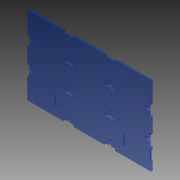
# Autodesk Inventor part: tableTop
Saved by Autodesk Inventor 2015 SP1 (Build 190203100, 203)
## iProperties
Created: 2015-04-09
Part Number: tableTop
Material: Generic
Document SubType Name: Modeling
Designer: Iain
Density: 1 g/cm^3
Appearance: Clear - Blue
Author: Iain
Autodesk Inventor part; units mm, degrees
(part 1 of 2)
sketch "Sketch1" plane through (0, 0, 0) normal (0, 1, 0) x (-1, 0, 0)
  line L0 (590, -375) -> (-590, -375)
  line L1 (-590, -375) -> (-590, 375)
  line L2 (-590, 375) -> (590, 375)
  line L3 (590, 375) -> (590, -375)
  point P0 (0, 0)
  point P1 (590, 0)
  point P2 (0, -375)
  dimension "d0" = 1180
  dimension "d1" = 750
  constraints: 8 end point, 2 midpoint, 2 parallel, 1 horizontal, 1 horizontal alignment, 1 perpendicular, 1 vertical alignment
  measures "d0" distance of L0.start L0.end
  measures "d1" distance of L2.end L0.start
extrude "Extrusion1" add sketch "Sketch1" along normal blind 18
sketch "Sketch2" plane through (0, 18, 0) normal (0, 1, 0) x (1, 0, 0)
  line L0 (590, 375) -> (-590, 375) projected
  line L1 (-590, 375) -> (-590, -375) projected
  line L2 (-590, -375) -> (590, -375) projected
  line L3 (590, -375) -> (590, 375) projected
  line L4 (-590, 175) -> (-572, 175)
  line L5 (-572, 175) -> (-572, 75)
  line L6 (-572, 75) -> (-590, 75)
  line L7 (-590, 75) -> (-590, 175)
  point P0 (0, 0)
  point P1 (-590, 125)
  point P2 (-590, 0)
  dimension "d4" = 18
  dimension "d5" = 100
  dimension "d6" = 250
  constraints: 8 end point, 2 midpoint, 2 parallel, 1 horizontal, 1 perpendicular, 1 vertical alignment
  measures "d4" distance of L4.start L4.end
  measures "d5" distance of L4.end L5.end
  measures "d6" distance of point (-590, 125) L0.end
extrude "Extrusion2" cut sketch "Sketch2" against normal blind 18 contours L4 L5 L6 L1
sketch "Sketch7" plane through (0, 18, 0) normal (0, 1, 0) x (1, 0, 0)
  line L0 (-590, 175) -> (-572, 175) projected
  line L1 (-572, 175) -> (-572, 75) projected
  line L2 (-572, 75) -> (-590, 75) projected
  line L3 (-590, 75) -> (-590, -375) projected
  line L4 (-590, -375) -> (590, -375) projected
  line L5 (590, -375) -> (590, 375) projected
  line L6 (590, 375) -> (-590, 375) projected
  line L7 (-590, 375) -> (-590, 175) projected
  line L8 (-590, 134) -> (-531, 134)
  line L9 (-531, 134) -> (-531, 116)
  line L10 (-531, 116) -> (-590, 116)
  line L11 (-590, 116) -> (-590, 134)
  point P0 (0, 0)
  point P1 (-590, 125)
  point P2 (-590, 275)
  point P3 (-531, 125)
  point P4 (-572, 125)
  dimension "d22" = 18
  dimension "d23" = 59
  constraints: 8 end point, 4 midpoint, 2 parallel, 1 horizontal, 1 horizontal alignment, 1 perpendicular, 1 vertical alignment
  measures "d22" distance of L8.end L9.end
  measures "d23" distance of L8.start L8.end
extrude "Extrusion6" cut sketch "Sketch7" against normal blind 18 contours L8 L9 L10 L1 | L1 L10 L11 L8
ref_plane "Work Plane1" through (0, 0, 375) normal (-1, 0, 0) x (0, 0, 1)
ref_plane "Work Plane2" through (-590, 0, 0) normal (0, 0, 1) x (1, 0, 0)
mirror "Mirror1" about plane through (0, 0, 375) normal (-1, 0, 0) of "Extrusion2", "Extrusion6"
mirror "Mirror7" about plane through (-590, 0, 0) normal (0, 0, 1) of "Extrusion2", "Extrusion6", "Mirror1"
sketch "Sketch3" plane through (0, 18, 0) normal (0, 1, 0) x (1, 0, 0)
  line L0 (590, 175) -> (590, 375) projected
  line L1 (590, 75) -> (572, 75) projected
  line L2 (572, 75) -> (572, 116) projected
  line L3 (572, 175) -> (590, 175) projected
  line L4 (590, 375) -> (-590, 375) projected
  line L5 (-590, 375) -> (-590, 175) projected
  line L6 (-590, 175) -> (-572, 175) projected
  line L7 (-572, 175) -> (-572, 134) projected
  line L8 (-572, 75) -> (-590, 75) projected
  line L9 (-590, -375) -> (590, -375) projected
  line L10 (-246.6667, 375) -> (-146.6667, 375)
  line L11 (-146.6667, 375) -> (-146.6667, 357)
  line L12 (-146.6667, 357) -> (-246.6667, 357)
  line L13 (-246.6667, 357) -> (-246.6667, 375)
  line L14 (590, -175) -> (572, -175) projected
  line L15 (572, -175) -> (572, -134) projected
  line L16 (572, -134) -> (531, -134) projected
  line L17 (531, -134) -> (531, -116) projected
  line L18 (531, -116) -> (572, -116) projected
  line L19 (572, -116) -> (572, -75) projected
  line L20 (572, -75) -> (590, -75) projected
  line L21 (590, -75) -> (590, 75) projected
  line L22 (572, 116) -> (531, 116) projected
  line L23 (531, 116) -> (531, 134) projected
  line L24 (531, 134) -> (572, 134) projected
  line L25 (572, 134) -> (572, 175) projected
  line L26 (-572, 134) -> (-531, 134) projected
  line L27 (-531, 134) -> (-531, 116) projected
  line L28 (-531, 116) -> (-572, 116) projected
  line L29 (-572, 116) -> (-572, 75) projected
  line L30 (-590, 75) -> (-590, -75) projected
  line L31 (-590, -75) -> (-572, -75) projected
  line L32 (-572, -75) -> (-572, -116) projected
  line L33 (-572, -116) -> (-531, -116) projected
  line L34 (-531, -116) -> (-531, -134) projected
  line L35 (-531, -134) -> (-572, -134) projected
  line L36 (-572, -134) -> (-572, -175) projected
  line L37 (-572, -175) -> (-590, -175) projected
  line L38 (-590, -175) -> (-590, -375) projected
  line L39 (590, -375) -> (590, -175) projected
  point P0 (0, 0)
  point P1 (-196.6667, 375)
  point P2 (0, 375)
  dimension "d9" = 18
  dimension "d10" = 100
  dimension "d11" = 393.3333
  constraints: 8 end point, 2 midpoint, 2 parallel, 1 horizontal, 1 horizontal alignment, 1 perpendicular
  measures "d9" distance of L10.end L11.end
  measures "d10" distance of L10.start L10.end
  measures "d11" distance of L4.end point (-196.667, 375)
extrude "Extrusion3" cut sketch "Sketch3" against normal blind 18 contours L11 L12 L13 L4
sketch "Sketch8" plane through (0, 18, 0) normal (0, 1, 0) x (1, 0, 0)
  line L0 (-146.6667, 375) -> (-146.6667, 357) projected
  line L1 (-146.6667, 357) -> (-246.6667, 357) projected
  line L2 (-246.6667, 357) -> (-246.6667, 375) projected
  line L3 (-246.6667, 375) -> (-590, 375) projected
  line L4 (-590, 375) -> (-590, 175) projected
  line L5 (-590, 175) -> (-572, 175) projected
  line L6 (-572, 175) -> (-572, 134) projected
  line L7 (-572, 134) -> (-531, 134) projected
  line L8 (-531, 134) -> (-531, 116) projected
  line L9 (-531, 116) -> (-572, 116) projected
  line L10 (-572, 116) -> (-572, 75) projected
  line L11 (-572, 75) -> (-590, 75) projected
  line L12 (-590, 75) -> (-590, -75) projected
  line L13 (-590, -75) -> (-572, -75) projected
  line L14 (-572, -75) -> (-572, -116) projected
  line L15 (-572, -116) -> (-531, -116) projected
  line L16 (-531, -116) -> (-531, -134) projected
  line L17 (-531, -134) -> (-572, -134) projected
  line L18 (-572, -134) -> (-572, -175) projected
  line L19 (-572, -175) -> (-590, -175) projected
  line L20 (-590, -175) -> (-590, -375) projected
  line L21 (-590, -375) -> (590, -375) projected
  line L22 (590, -375) -> (590, -175) projected
  line L23 (590, -175) -> (572, -175) projected
  line L24 (572, -175) -> (572, -134) projected
  line L25 (572, -134) -> (531, -134) projected
  line L26 (531, -134) -> (531, -116) projected
  line L27 (531, -116) -> (572, -116) projected
  line L28 (572, -116) -> (572, -75) projected
  line L29 (572, -75) -> (590, -75) projected
  line L30 (590, -75) -> (590, 75) projected
  line L31 (590, 75) -> (572, 75) projected
  line L32 (572, 75) -> (572, 116) projected
  line L33 (572, 116) -> (531, 116) projected
  line L34 (531, 116) -> (531, 134) projected
  line L35 (531, 134) -> (572, 134) projected
  line L36 (572, 134) -> (572, 175) projected
  line L37 (572, 175) -> (590, 175) projected
  line L38 (590, 175) -> (590, 375) projected
  line L39 (590, 375) -> (-146.6667, 375) projected
  line L40 (-205.6667, 375) -> (-187.6667, 375)
  line L41 (-187.6667, 375) -> (-187.6667, 316)
  line L42 (-187.6667, 316) -> (-205.6667, 316)
  line L43 (-205.6667, 316) -> (-205.6667, 375)
  point P0 (0, 0)
  point P1 (-196.6667, 375)
  point P2 (-418.3333, 375)
  point P3 (-196.6667, 316)
  point P4 (-196.6667, 357)
  dimension "d26" = 18
  dimension "d27" = 59
  constraints: 8 end point, 4 midpoint, 2 parallel, 1 horizontal, 1 horizontal alignment, 1 perpendicular, 1 vertical alignment
  measures "d26" distance of L40.start L40.end
  measures "d27" distance of L40.end L41.end
extrude "Extrusion7" cut sketch "Sketch8" against normal blind 18 contours L41 L42 L43 L1 | L1 L43 L40 L41
mirror "Mirror3" about plane through (0, 0, 375) normal (-1, 0, 0) of "Extrusion3", "Extrusion7"
mirror "Mirror8" about plane through (-590, 0, 0) normal (0, 0, 1) of "Extrusion3", "Extrusion7", "Mirror3"
sketch "Sketch4" plane through (0, 18, 0) normal (0, 1, 0) x (1, 0, 0)
  line L0 (-246.6667, 134) -> (-146.6667, 134)
  line L1 (-146.6667, 134) -> (-146.6667, 116)
  line L2 (-146.6667, 116) -> (-246.6667, 116)
  line L3 (-246.6667, 116) -> (-246.6667, 134)
  line L4 (-590, -375) -> (-246.6667, -375) projected
  line L5 (590, -375) -> (590, -175) projected
  line L6 (590, 75) -> (572, 75) projected
  line L7 (572, 75) -> (572, 116) projected
  line L8 (572, 175) -> (590, 175) projected
  line L9 (590, 175) -> (590, 375) projected
  line L10 (590, 375) -> (246.6667, 375) projected
  line L11 (246.6667, 375) -> (246.6667, 357) projected
  line L12 (246.6667, 357) -> (205.6667, 357) projected
  line L13 (146.6667, 357) -> (146.6667, 375) projected
  line L14 (146.6667, 375) -> (-146.6667, 375) projected
  line L15 (-146.6667, 375) -> (-146.6667, 357) projected
  line L16 (-146.6667, 357) -> (-187.6667, 357) projected
  line L17 (-246.6667, 357) -> (-246.6667, 375) projected
  line L18 (-246.6667, 375) -> (-590, 375) projected
  line L19 (-590, 375) -> (-590, 175) projected
  line L20 (-590, 175) -> (-572, 175) projected
  line L21 (-572, 175) -> (-572, 134) projected
  line L22 (-572, 75) -> (-590, 75) projected
  line L23 (590, -175) -> (572, -175) projected
  line L24 (572, -175) -> (572, -134) projected
  line L25 (572, -134) -> (531, -134) projected
  line L26 (531, -134) -> (531, -116) projected
  line L27 (531, -116) -> (572, -116) projected
  line L28 (572, -116) -> (572, -75) projected
  line L29 (572, -75) -> (590, -75) projected
  line L30 (572, 116) -> (531, 116) projected
  line L31 (531, 116) -> (531, 134) projected
  line L32 (531, 134) -> (572, 134) projected
  line L33 (572, 134) -> (572, 175) projected
  line L34 (205.6667, 357) -> (205.6667, 316) projected
  line L35 (205.6667, 316) -> (187.6667, 316) projected
  line L36 (187.6667, 316) -> (187.6667, 357) projected
  line L37 (187.6667, 357) -> (146.6667, 357) projected
  line L38 (-187.6667, 357) -> (-187.6667, 316) projected
  line L39 (-187.6667, 316) -> (-205.6667, 316) projected
  line L40 (-205.6667, 316) -> (-205.6667, 357) projected
  line L41 (-205.6667, 357) -> (-246.6667, 357) projected
  line L42 (-572, 134) -> (-531, 134) projected
  line L43 (-531, 134) -> (-531, 116) projected
  line L44 (-531, 116) -> (-572, 116) projected
  line L45 (-572, 116) -> (-572, 75) projected
  line L46 (-590, 75) -> (-590, -75) projected
  line L47 (-590, -75) -> (-572, -75) projected
  line L48 (-572, -75) -> (-572, -116) projected
  line L49 (-572, -116) -> (-531, -116) projected
  line L50 (-531, -116) -> (-531, -134) projected
  line L51 (-531, -134) -> (-572, -134) projected
  line L52 (-572, -134) -> (-572, -175) projected
  line L53 (-572, -175) -> (-590, -175) projected
  line L54 (246.6667, -357) -> (246.6667, -375) projected
  line L55 (246.6667, -375) -> (590, -375) projected
  line L56 (-246.6667, -375) -> (-246.6667, -357) projected
  line L57 (-246.6667, -357) -> (-205.6667, -357) projected
  line L58 (-205.6667, -357) -> (-205.6667, -316) projected
  line L59 (-205.6667, -316) -> (-187.6667, -316) projected
  line L60 (-187.6667, -316) -> (-187.6667, -357) projected
  line L61 (-187.6667, -357) -> (-146.6667, -357) projected
  line L62 (-146.6667, -357) -> (-146.6667, -375) projected
  line L63 (-146.6667, -375) -> (146.6667, -375) projected
  line L64 (146.6667, -375) -> (146.6667, -357) projected
  line L65 (146.6667, -357) -> (187.6667, -357) projected
  line L66 (187.6667, -357) -> (187.6667, -316) projected
  line L67 (187.6667, -316) -> (205.6667, -316) projected
  line L68 (205.6667, -316) -> (205.6667, -357) projected
  line L69 (205.6667, -357) -> (246.6667, -357) projected
  line L70 (590, -75) -> (590, 75) projected
  line L71 (-590, -175) -> (-590, -375) projected
  point P0 (0, 0)
  point P1 (-196.6667, 134)
  point P2 (-167.1667, 357)
  point P3 (-246.6667, 125)
  point P4 (-572, 154.5)
  point P5 (-531, 125)
  point P6 (-196.6667, 316)
  dimension "d14" = 18
  dimension "d15" = 100
  constraints: 8 end point, 6 midpoint, 2 parallel, 1 horizontal, 1 horizontal alignment, 1 perpendicular, 1 vertical alignment
  measures "d14" distance of L0.end L1.end
  measures "d15" distance of L0.start L0.end
extrude "Extrusion4" cut sketch "Sketch4" against normal blind 18 contours L0 L1 L2 L3
sketch "Sketch5" plane through (0, 18, 0) normal (0, 1, 0) x (1, 0, 0)
  line L0 (-246.6667, 116) -> (-246.6667, 134) projected
  line L1 (-246.6667, 134) -> (-146.6667, 134) projected
  line L2 (-146.6667, 134) -> (-146.6667, 116) projected
  line L3 (-146.6667, 116) -> (-246.6667, 116) projected
  line L4 (-590, -375) -> (-246.6667, -375) projected
  line L5 (590, -375) -> (590, -175) projected
  line L6 (590, 75) -> (572, 75) projected
  line L7 (572, 75) -> (572, 116) projected
  line L8 (572, 175) -> (590, 175) projected
  line L9 (590, 175) -> (590, 375) projected
  line L10 (590, 375) -> (246.6667, 375) projected
  line L11 (246.6667, 375) -> (246.6667, 357) projected
  line L12 (246.6667, 357) -> (205.6667, 357) projected
  line L13 (146.6667, 357) -> (146.6667, 375) projected
  line L14 (146.6667, 375) -> (-146.6667, 375) projected
  line L15 (-146.6667, 375) -> (-146.6667, 357) projected
  line L16 (-146.6667, 357) -> (-187.6667, 357) projected
  line L17 (-246.6667, 357) -> (-246.6667, 375) projected
  line L18 (-246.6667, 375) -> (-590, 375) projected
  line L19 (-590, 375) -> (-590, 175) projected
  line L20 (-590, 175) -> (-572, 175) projected
  line L21 (-572, 175) -> (-572, 134) projected
  line L22 (-572, 75) -> (-590, 75) projected
  line L23 (-205.6667, 175) -> (-187.6667, 175)
  line L24 (-187.6667, 175) -> (-187.6667, 75)
  line L25 (-187.6667, 75) -> (-205.6667, 75)
  line L26 (-205.6667, 75) -> (-205.6667, 175)
  line L27 (590, -175) -> (572, -175) projected
  line L28 (572, -175) -> (572, -134) projected
  line L29 (572, -134) -> (531, -134) projected
  line L30 (531, -134) -> (531, -116) projected
  line L31 (531, -116) -> (572, -116) projected
  line L32 (572, -116) -> (572, -75) projected
  line L33 (572, -75) -> (590, -75) projected
  line L34 (572, 116) -> (531, 116) projected
  line L35 (531, 116) -> (531, 134) projected
  line L36 (531, 134) -> (572, 134) projected
  line L37 (572, 134) -> (572, 175) projected
  line L38 (205.6667, 357) -> (205.6667, 316) projected
  line L39 (205.6667, 316) -> (187.6667, 316) projected
  line L40 (187.6667, 316) -> (187.6667, 357) projected
  line L41 (187.6667, 357) -> (146.6667, 357) projected
  line L42 (-187.6667, 357) -> (-187.6667, 316) projected
  line L43 (-187.6667, 316) -> (-205.6667, 316) projected
  line L44 (-205.6667, 316) -> (-205.6667, 357) projected
  line L45 (-205.6667, 357) -> (-246.6667, 357) projected
  line L46 (-572, 134) -> (-531, 134) projected
  line L47 (-531, 134) -> (-531, 116) projected
  line L48 (-531, 116) -> (-572, 116) projected
  line L49 (-572, 116) -> (-572, 75) projected
  line L50 (-590, 75) -> (-590, -75) projected
  line L51 (-590, -75) -> (-572, -75) projected
  line L52 (-572, -75) -> (-572, -116) projected
  line L53 (-572, -116) -> (-531, -116) projected
  line L54 (-531, -116) -> (-531, -134) projected
  line L55 (-531, -134) -> (-572, -134) projected
  line L56 (-572, -134) -> (-572, -175) projected
  line L57 (-572, -175) -> (-590, -175) projected
  line L58 (246.6667, -357) -> (246.6667, -375) projected
  line L59 (-246.6667, -375) -> (-246.6667, -357) projected
  line L60 (-246.6667, -357) -> (-205.6667, -357) projected
  line L61 (-205.6667, -357) -> (-205.6667, -316) projected
  line L62 (-205.6667, -316) -> (-187.6667, -316) projected
  line L63 (-187.6667, -316) -> (-187.6667, -357) projected
  line L64 (-187.6667, -357) -> (-146.6667, -357) projected
  line L65 (-146.6667, -357) -> (-146.6667, -375) projected
  line L66 (-146.6667, -375) -> (146.6667, -375) projected
  line L67 (146.6667, -375) -> (146.6667, -357) projected
  line L68 (146.6667, -357) -> (187.6667, -357) projected
  line L69 (187.6667, -357) -> (187.6667, -316) projected
  line L70 (187.6667, -316) -> (205.6667, -316) projected
  line L71 (205.6667, -316) -> (205.6667, -357) projected
  line L72 (205.6667, -357) -> (246.6667, -357) projected
  line L73 (246.6667, -375) -> (590, -375) projected
  line L74 (590, -75) -> (590, 75) projected
  line L75 (-590, -175) -> (-590, -375) projected
  point P0 (0, 0)
  point P1 (-205.6667, 125)
  point P2 (-572, 154.5)
  point P3 (-167.1667, 357)
  point P4 (-196.6667, 175)
  point P5 (-531, 125)
  point P6 (-196.6667, 316)
  dimension "d18" = 18
  dimension "d19" = 100
  constraints: 8 end point, 6 midpoint, 2 parallel, 1 horizontal, 1 horizontal alignment, 1 perpendicular, 1 vertical alignment
  measures "d18" distance of L23.start L23.end
  measures "d19" distance of L25.end L23.start
extrude "Extrusion5" cut sketch "Sketch5" against normal blind 18 contours L26 L1 L24 L3 | L3 L24 L25 L26 | L26 L23 L24 L1
mirror "Mirror5" about plane through (0, 0, 375) normal (-1, 0, 0) of "Extrusion4", "Extrusion5"
mirror "Mirror9" about plane through (-590, 0, 0) normal (0, 0, 1) of "Extrusion4", "Extrusion5", "Mirror5"
sketch "Sketch9" plane through (0, 18, 0) normal (0, 1, 0) x (1, 0, 0)
  line L0 (246.6667, -116) -> (246.6667, -134) projected
  line L1 (246.6667, -134) -> (205.6667, -134) projected
  line L2 (205.6667, -134) -> (205.6667, -175) projected
  line L3 (205.6667, -175) -> (187.6667, -175) projected
  line L4 (187.6667, -175) -> (187.6667, -134) projected
  line L5 (187.6667, -134) -> (146.6667, -134) projected
  line L6 (146.6667, -134) -> (146.6667, -116) projected
  line L7 (146.6667, -116) -> (187.6667, -116) projected
  line L8 (187.6667, -116) -> (187.6667, -75) projected
  line L9 (187.6667, -75) -> (205.6667, -75) projected
  line L10 (205.6667, -75) -> (205.6667, -116) projected
  line L11 (205.6667, -116) -> (246.6667, -116) projected
  line L12 (-246.6667, -134) -> (-246.6667, -116) projected
  line L13 (-246.6667, -116) -> (-205.6667, -116) projected
  line L14 (-205.6667, -116) -> (-205.6667, -75) projected
  line L15 (-205.6667, -75) -> (-187.6667, -75) projected
  line L16 (-187.6667, -75) -> (-187.6667, -116) projected
  line L17 (-187.6667, -116) -> (-146.6667, -116) projected
  line L18 (-146.6667, -116) -> (-146.6667, -134) projected
  line L19 (-146.6667, -134) -> (-187.6667, -134) projected
  line L20 (-187.6667, -134) -> (-187.6667, -175) projected
  line L21 (-187.6667, -175) -> (-205.6667, -175) projected
  line L22 (-205.6667, -175) -> (-205.6667, -134) projected
  line L23 (-205.6667, -134) -> (-246.6667, -134) projected
  line L24 (246.6667, 134) -> (246.6667, 116) projected
  line L25 (246.6667, 116) -> (205.6667, 116) projected
  line L26 (205.6667, 116) -> (205.6667, 75) projected
  line L27 (205.6667, 75) -> (187.6667, 75) projected
  line L28 (187.6667, 75) -> (187.6667, 116) projected
  line L29 (187.6667, 116) -> (146.6667, 116) projected
  line L30 (146.6667, 116) -> (146.6667, 134) projected
  line L31 (146.6667, 134) -> (187.6667, 134) projected
  line L32 (187.6667, 134) -> (187.6667, 175) projected
  line L33 (187.6667, 175) -> (205.6667, 175) projected
  line L34 (205.6667, 175) -> (205.6667, 134) projected
  line L35 (205.6667, 134) -> (246.6667, 134) projected
  line L36 (-205.6667, 75) -> (-205.6667, 116) projected
  line L37 (-205.6667, 116) -> (-246.6667, 116) projected
  line L38 (-246.6667, 116) -> (-246.6667, 134) projected
  line L39 (-246.6667, 134) -> (-205.6667, 134) projected
  line L40 (-205.6667, 134) -> (-205.6667, 175) projected
  line L41 (-205.6667, 175) -> (-187.6667, 175) projected
  line L42 (-187.6667, 175) -> (-187.6667, 134) projected
  line L43 (-187.6667, 134) -> (-146.6667, 134) projected
  line L44 (-146.6667, 134) -> (-146.6667, 116) projected
  line L45 (-146.6667, 116) -> (-187.6667, 116) projected
  line L46 (-187.6667, 116) -> (-187.6667, 75) projected
  line L47 (-187.6667, 75) -> (-205.6667, 75) projected
  line L48 (246.6667, -357) -> (246.6667, -375) projected
  line L49 (246.6667, -375) -> (590, -375) projected
  line L50 (590, -375) -> (590, -175) projected
  line L51 (590, -175) -> (572, -175) projected
  line L52 (572, -175) -> (572, -134) projected
  line L53 (572, -134) -> (531, -134) projected
  line L54 (531, -134) -> (531, -116) projected
  line L55 (531, -116) -> (572, -116) projected
  line L56 (572, -116) -> (572, -75) projected
  line L57 (572, -75) -> (590, -75) projected
  line L58 (590, -75) -> (590, 75) projected
  line L59 (590, 75) -> (572, 75) projected
  line L60 (572, 75) -> (572, 116) projected
  line L61 (572, 116) -> (531, 116) projected
  line L62 (531, 116) -> (531, 134) projected
  line L63 (531, 134) -> (572, 134) projected
  line L64 (572, 134) -> (572, 175) projected
  line L65 (572, 175) -> (590, 175) projected
  line L66 (590, 175) -> (590, 375) projected
  line L67 (590, 375) -> (246.6667, 375) projected
  line L68 (246.6667, 375) -> (246.6667, 357) projected
  line L69 (246.6667, 357) -> (205.6667, 357) projected
  line L70 (205.6667, 357) -> (205.6667, 316) projected
  line L71 (205.6667, 316) -> (187.6667, 316) projected
  line L72 (187.6667, 316) -> (187.6667, 357) projected
  line L73 (187.6667, 357) -> (146.6667, 357) projected
  line L74 (146.6667, 357) -> (146.6667, 375) projected
  line L75 (146.6667, 375) -> (-146.6667, 375) projected
  line L76 (-146.6667, 375) -> (-146.6667, 357) projected
  line L77 (-146.6667, 357) -> (-187.6667, 357) projected
  line L78 (-187.6667, 357) -> (-187.6667, 316) projected
  line L79 (-187.6667, 316) -> (-205.6667, 316) projected
  line L80 (-205.6667, 316) -> (-205.6667, 357) projected
  line L81 (-205.6667, 357) -> (-246.6667, 357) projected
  line L82 (-246.6667, 357) -> (-246.6667, 375) projected
  line L83 (-246.6667, 375) -> (-590, 375) projected
  line L84 (-590, 375) -> (-590, 175) projected
  line L85 (-590, 175) -> (-572, 175) projected
  line L86 (-572, 175) -> (-572, 134) projected
  line L87 (-572, 134) -> (-531, 134) projected
  line L88 (-531, 134) -> (-531, 116) projected
  line L89 (-531, 116) -> (-572, 116) projected
  line L90 (-572, 116) -> (-572, 75) projected
  line L91 (-572, 75) -> (-590, 75) projected
  line L92 (-590, 75) -> (-590, -75) projected
  line L93 (-590, -75) -> (-572, -75) projected
  line L94 (-572, -75) -> (-572, -116) projected
  line L95 (-572, -116) -> (-531, -116) projected
  line L96 (-531, -116) -> (-531, -134) projected
  line L97 (-531, -134) -> (-572, -134) projected
  line L98 (-572, -134) -> (-572, -175) projected
  line L99 (-572, -175) -> (-590, -175) projected
  line L100 (-590, -175) -> (-590, -375) projected
  line L101 (-590, -375) -> (-246.6667, -375) projected
  line L102 (-246.6667, -375) -> (-246.6667, -357) projected
  line L103 (-246.6667, -357) -> (-205.6667, -357) projected
  line L104 (-205.6667, -357) -> (-205.6667, -316) projected
  line L105 (-205.6667, -316) -> (-187.6667, -316) projected
  line L106 (-187.6667, -316) -> (-187.6667, -357) projected
  line L107 (-187.6667, -357) -> (-146.6667, -357) projected
  line L108 (-146.6667, -357) -> (-146.6667, -375) projected
  line L109 (-146.6667, -375) -> (146.6667, -375) projected
  line L110 (146.6667, -375) -> (146.6667, -357) projected
  line L111 (146.6667, -357) -> (187.6667, -357) projected
  line L112 (187.6667, -357) -> (187.6667, -316) projected
  line L113 (187.6667, -316) -> (205.6667, -316) projected
  line L114 (205.6667, -316) -> (205.6667, -357) projected
  line L115 (205.6667, -357) -> (246.6667, -357) projected
  line L116 (-590, 375) -> (590, 375) construction
  line L117 (590, 375) -> (590, 125) construction
  line L118 (590, 125) -> (-590, 125) construction
  line L119 (-590, 125) -> (-590, 375) construction
  line L120 (146.6667, 375) -> (-146.6667, 375) construction
  line L121 (-590, 291.6667) -> (-572, 291.6667)
  line L122 (-572, 291.6667) -> (-572, 208.3333)
  line L123 (-572, 208.3333) -> (-590, 208.3333)
  line L124 (-590, 208.3333) -> (-590, 291.6667)
  point P0 (0, 0)
  point P1 (0, 375)
  point P2 (0, 375)
  point P3 (0, 375)
  point P4 (-590, 250)
  point P5 (-590, 250)
  dimension "d30" = 250
  dimension "d31" = 1180
  dimension "d32" = 18
  dimension "d33" = 83.3333
  constraints: 16 end point, 5 midpoint, 4 coincident, 4 parallel, 2 horizontal, 2 perpendicular
  measures "d30" distance of L116.end L117.end
  measures "d31" distance of L117.end L118.end
  measures "d32" distance of L121.start L121.end
  measures "d33" distance of L121.end L122.end
sketch "Sketch10" plane through (0, 18, 0) normal (0, 1, 0) x (1, 0, 0)
  line L0 (-590, 125) -> (-590, 375) construction
  line L1 (590, 125) -> (-590, 125) construction
  line L2 (-590, 375) -> (590, 375) construction
  line L3 (590, 375) -> (590, 125) construction
  line L4 (-336.7778, 291.6667) -> (-318.7778, 291.6667)
  line L5 (-318.7778, 291.6667) -> (-318.7778, 208.3333)
  line L6 (-318.7778, 208.3333) -> (-336.7778, 208.3333)
  line L7 (-336.7778, 208.3333) -> (-336.7778, 291.6667)
  line L8 (-336.7778, 291.6667) -> (-327.7778, 291.6667) construction
  point P0 (0, 0)
  point P1 (-318.7778, 250)
  point P2 (-590, 250)
  point P3 (-332.2778, 291.6667)
  dimension "d36" = 83.3333
  dimension "d37" = 18
  dimension "d38" = 9
  dimension "d39" = 262.2222
  constraints: 10 end point, 4 midpoint, 2 horizontal, 2 horizontal alignment, 2 parallel, 1 coincident, 1 perpendicular
  measures "d36" distance of L4.end L5.end
  measures "d37" distance of L4.start L4.end
  measures "d38" distance of L8.start L8.end
  measures "d39" horizontal distance of point (-590, 250) L8.end
extrude "Extrusion8" cut sketch "Sketch9" against normal blind 9 contours L84 L121 L122 L123
extrude "Extrusion9" cut sketch "Sketch10" against normal blind 9
mirror "Mirror10" about plane through (0, 0, 375) normal (-1, 0, 0) of "Extrusion8", "Extrusion9"
sketch "Sketch11" plane through (0, 18, 0) normal (0, 1, 0) x (1, 0, 0)
  line L0 (246.6667, -116) -> (246.6667, -134) projected
  line L1 (246.6667, -134) -> (205.6667, -134) projected
  line L2 (205.6667, -134) -> (205.6667, -175) projected
  line L3 (205.6667, -175) -> (187.6667, -175) projected
  line L4 (187.6667, -175) -> (187.6667, -134) projected
  line L5 (187.6667, -134) -> (146.6667, -134) projected
  line L6 (146.6667, -134) -> (146.6667, -116) projected
  line L7 (146.6667, -116) -> (187.6667, -116) projected
  line L8 (187.6667, -116) -> (187.6667, -75) projected
  line L9 (187.6667, -75) -> (205.6667, -75) projected
  line L10 (205.6667, -75) -> (205.6667, -116) projected
  line L11 (205.6667, -116) -> (246.6667, -116) projected
  line L12 (-246.6667, -134) -> (-246.6667, -116) projected
  line L13 (-246.6667, -116) -> (-205.6667, -116) projected
  line L14 (-205.6667, -116) -> (-205.6667, -75) projected
  line L15 (-205.6667, -75) -> (-187.6667, -75) projected
  line L16 (-187.6667, -75) -> (-187.6667, -116) projected
  line L17 (-187.6667, -116) -> (-146.6667, -116) projected
  line L18 (-146.6667, -116) -> (-146.6667, -134) projected
  line L19 (-146.6667, -134) -> (-187.6667, -134) projected
  line L20 (-187.6667, -134) -> (-187.6667, -175) projected
  line L21 (-187.6667, -175) -> (-205.6667, -175) projected
  line L22 (-205.6667, -175) -> (-205.6667, -134) projected
  line L23 (-205.6667, -134) -> (-246.6667, -134) projected
  line L24 (246.6667, 134) -> (246.6667, 116) projected
  line L25 (246.6667, 116) -> (205.6667, 116) projected
  line L26 (205.6667, 116) -> (205.6667, 75) projected
  line L27 (205.6667, 75) -> (187.6667, 75) projected
  line L28 (187.6667, 75) -> (187.6667, 116) projected
  line L29 (187.6667, 116) -> (146.6667, 116) projected
  line L30 (146.6667, 116) -> (146.6667, 134) projected
  line L31 (146.6667, 134) -> (187.6667, 134) projected
  line L32 (187.6667, 134) -> (187.6667, 175) projected
  line L33 (187.6667, 175) -> (205.6667, 175) projected
  line L34 (205.6667, 175) -> (205.6667, 134) projected
  line L35 (205.6667, 134) -> (246.6667, 134) projected
  line L36 (-205.6667, 75) -> (-205.6667, 116) projected
  line L37 (-205.6667, 116) -> (-246.6667, 116) projected
  line L38 (-246.6667, 116) -> (-246.6667, 134) projected
  line L39 (-246.6667, 134) -> (-205.6667, 134) projected
  line L40 (-205.6667, 134) -> (-205.6667, 175) projected
  line L41 (-205.6667, 175) -> (-187.6667, 175) projected
  line L42 (-187.6667, 175) -> (-187.6667, 134) projected
  line L43 (-187.6667, 134) -> (-146.6667, 134) projected
  line L44 (-146.6667, 134) -> (-146.6667, 116) projected
  line L45 (-146.6667, 116) -> (-187.6667, 116) projected
  line L46 (-187.6667, 116) -> (-187.6667, 75) projected
  line L47 (-187.6667, 75) -> (-205.6667, 75) projected
  line L48 (590, 208.3333) -> (572, 208.3333) projected
  line L49 (572, 208.3333) -> (572, 291.6667) projected
  line L50 (572, 291.6667) -> (590, 291.6667) projected
  line L51 (590, 291.6667) -> (590, 375) projected
  line L52 (590, 375) -> (246.6667, 375) projected
  line L53 (246.6667, 375) -> (246.6667, 357) projected
  line L54 (246.6667, 357) -> (205.6667, 357) projected
  line L55 (205.6667, 357) -> (205.6667, 316) projected
  line L56 (205.6667, 316) -> (187.6667, 316) projected
  line L57 (187.6667, 316) -> (187.6667, 357) projected
  line L58 (187.6667, 357) -> (146.6667, 357) projected
  line L59 (146.6667, 357) -> (146.6667, 375) projected
  line L60 (146.6667, 375) -> (-146.6667, 375) projected
  line L61 (-146.6667, 375) -> (-146.6667, 357) projected
  line L62 (-146.6667, 357) -> (-187.6667, 357) projected
  line L63 (-187.6667, 357) -> (-187.6667, 316) projected
  line L64 (-187.6667, 316) -> (-205.6667, 316) projected
  line L65 (-205.6667, 316) -> (-205.6667, 357) projected
  line L66 (-205.6667, 357) -> (-246.6667, 357) projected
  line L67 (-246.6667, 357) -> (-246.6667, 375) projected
  line L68 (-246.6667, 375) -> (-590, 375) projected
  line L69 (-590, 375) -> (-590, 291.6667) projected
  line L70 (-590, 291.6667) -> (-572, 291.6667) projected
  line L71 (-572, 291.6667) -> (-572, 208.3333) projected
  line L72 (-572, 208.3333) -> (-590, 208.3333) projected
  line L73 (-590, 208.3333) -> (-590, 175) projected
  line L74 (-590, 175) -> (-572, 175) projected
  line L75 (-572, 175) -> (-572, 134) projected
  line L76 (-572, 134) -> (-531, 134) projected
  line L77 (-531, 134) -> (-531, 116) projected
  line L78 (-531, 116) -> (-572, 116) projected
  line L79 (-572, 116) -> (-572, 75) projected
  line L80 (-572, 75) -> (-590, 75) projected
  line L81 (-590, 75) -> (-590, -75) projected
  line L82 (-590, -75) -> (-572, -75) projected
  line L83 (-572, -75) -> (-572, -116) projected
  line L84 (-572, -116) -> (-531, -116) projected
  line L85 (-531, -116) -> (-531, -134) projected
  line L86 (-531, -134) -> (-572, -134) projected
  line L87 (-572, -134) -> (-572, -175) projected
  line L88 (-572, -175) -> (-590, -175) projected
  line L89 (-590, -175) -> (-590, -375) projected
  line L90 (-590, -375) -> (-246.6667, -375) projected
  line L91 (-246.6667, -375) -> (-246.6667, -357) projected
  line L92 (-246.6667, -357) -> (-205.6667, -357) projected
  line L93 (-205.6667, -357) -> (-205.6667, -316) projected
  line L94 (-205.6667, -316) -> (-187.6667, -316) projected
  line L95 (-187.6667, -316) -> (-187.6667, -357) projected
  line L96 (-187.6667, -357) -> (-146.6667, -357) projected
  line L97 (-146.6667, -357) -> (-146.6667, -375) projected
  line L98 (-146.6667, -375) -> (146.6667, -375) projected
  line L99 (146.6667, -375) -> (146.6667, -357) projected
  line L100 (146.6667, -357) -> (187.6667, -357) projected
  line L101 (187.6667, -357) -> (187.6667, -316) projected
  line L102 (187.6667, -316) -> (205.6667, -316) projected
  line L103 (205.6667, -316) -> (205.6667, -357) projected
  line L104 (205.6667, -357) -> (246.6667, -357) projected
  line L105 (246.6667, -357) -> (246.6667, -375) projected
  line L106 (246.6667, -375) -> (590, -375) projected
  line L107 (590, -375) -> (590, -175) projected
  line L108 (590, -175) -> (572, -175) projected
  line L109 (572, -175) -> (572, -134) projected
  line L110 (572, -134) -> (531, -134) projected
  line L111 (531, -134) -> (531, -116) projected
  line L112 (531, -116) -> (572, -116) projected
  line L113 (572, -116) -> (572, -75) projected
  line L114 (572, -75) -> (590, -75) projected
  line L115 (590, -75) -> (590, 75) projected
  line L116 (590, 75) -> (572, 75) projected
  line L117 (572, 75) -> (572, 116) projected
  line L118 (572, 116) -> (531, 116) projected
  line L119 (531, 116) -> (531, 134) projected
  line L120 (531, 134) -> (572, 134) projected
  line L121 (572, 134) -> (572, 175) projected
  line L122 (572, 175) -> (590, 175) projected
  line L123 (590, 175) -> (590, 208.3333) projected
  line L124 (-336.7778, 208.3333) -> (-336.7778, 291.6667) projected
  line L125 (-336.7778, 291.6667) -> (-318.7778, 291.6667) projected
  line L126 (-318.7778, 291.6667) -> (-318.7778, 208.3333) projected
  line L127 (-318.7778, 208.3333) -> (-336.7778, 208.3333) projected
  line L128 (336.7778, 291.6667) -> (336.7778, 208.3333) projected
  line L129 (336.7778, 208.3333) -> (318.7778, 208.3333) projected
  line L130 (318.7778, 208.3333) -> (318.7778, 291.6667) projected
  line L131 (318.7778, 291.6667) -> (336.7778, 291.6667) projected
  point P0 (0, 0)
  point P1 (-572, 171.825)
  point P2 (-534.175, 134)
  point P3 (-572, 154.5)
  point P4 (-551.5, 134)
  dimension "d44" = 3.175
  dimension "d45" = 3.175
  constraints: 2 midpoint, 1 horizontal alignment, 1 vertical alignment
  measures "d44" distance from line of point (-572, 171.825) L74
  measures "d45" distance from line of L77 point (-534.175, 134)
hole "Hole1" at (-572, 18, -171.825) at (-534.175, 18, -134) direction (0, -1, 0) diameter 6.35 end through all
ref_plane "Work Plane4" through (-572, 0, -125) normal (0, 0, 1) x (1, 0, 0)
mirror "Mirror11" about plane through (-572, 0, -125) normal (0, 0, 1) of "Hole1"
mirror "Mirror12" about plane through (-590, 0, 0) normal (0, 0, 1) of "Hole1", "Mirror11"
mirror "Mirror13" about plane through (0, 0, 375) normal (-1, 0, 0) of "Hole1", "Mirror11", "Mirror12"
sketch "Sketch12" plane through (0, 18, 0) normal (0, 1, 0) x (1, 0, 0)
  line L0 (-246.6667, 357) -> (-246.6667, 375) projected
  line L1 (-187.6667, 316) -> (-205.6667, 316) projected
  point P0 (0, 0)
  point P1 (-243.4917, 357)
  point P2 (-205.6667, 319.175)
  dimension "d53" = 3.175
  dimension "d54" = 3.175
  constraints: 1 horizontal alignment, 1 vertical alignment
  measures "d53" distance from line of L0 point (-243.492, 357)
  measures "d54" distance from line of L1 point (-205.667, 319.175)
hole "Hole2" at (-243.4917, 18, -357) at (-205.6667, 18, -319.175) direction (0, -1, 0) diameter 6.35 end through all
ref_plane "Work Plane5" through (-196.6667, 0, -357) normal (1, 0, 0) x (0, 0, -1)
mirror "Mirror14" about plane through (-196.6667, 0, -357) normal (1, 0, 0) of "Hole2"
mirror "Mirror15" about plane through (0, 0, 375) normal (-1, 0, 0) of "Hole2", "Mirror14"
mirror "Mirror16" about plane through (-590, 0, 0) normal (0, 0, 1) of "Hole2", "Mirror14", "Mirror15"
sketch "Sketch13" plane through (0, 18, 0) normal (0, 1, 0) x (1, 0, 0)
  arc A0 (153.0167, -357) -> (146.6667, -357) centre (149.8417, -357) ccw projected
  line L0 (153.0167, -357) -> (187.6667, -357) projected
  line L1 (187.6667, -357) -> (187.6667, -322.35) projected
  arc A1 (187.6667, -316) -> (187.6667, -322.35) centre (187.6667, -319.175) ccw projected
  line L2 (187.6667, -316) -> (205.6667, -316) projected
  arc A2 (205.6667, -322.35) -> (205.6667, -316) centre (205.6667, -319.175) ccw projected
  line L3 (205.6667, -322.35) -> (205.6667, -357) projected
  line L4 (205.6667, -357) -> (240.3167, -357) projected
  arc A3 (246.6667, -357) -> (240.3167, -357) centre (243.4917, -357) ccw projected
  line L5 (246.6667, -357) -> (246.6667, -375) projected
  line L6 (246.6667, -375) -> (590, -375) projected
  line L7 (590, -375) -> (590, -175) projected
  line L8 (590, -175) -> (572, -175) projected
  arc A4 (572, -168.65) -> (572, -175) centre (572, -171.825) ccw projected
  line L9 (572, -168.65) -> (572, -134) projected
  line L10 (572, -134) -> (537.35, -134) projected
  arc A5 (531, -134) -> (537.35, -134) centre (534.175, -134) ccw projected
  line L11 (531, -134) -> (531, -116) projected
  arc A6 (537.35, -116) -> (531, -116) centre (534.175, -116) ccw projected
  line L12 (537.35, -116) -> (572, -116) projected
  line L13 (572, -116) -> (572, -81.35) projected
  arc A7 (572, -75) -> (572, -81.35) centre (572, -78.175) ccw projected
  line L14 (572, -75) -> (590, -75) projected
  line L15 (590, -75) -> (590, 75) projected
  line L16 (590, 75) -> (572, 75) projected
  arc A8 (572, 81.35) -> (572, 75) centre (572, 78.175) ccw projected
  line L17 (572, 81.35) -> (572, 116) projected
  line L18 (572, 116) -> (537.35, 116) projected
  arc A9 (531, 116) -> (537.35, 116) centre (534.175, 116) ccw projected
  line L19 (531, 116) -> (531, 134) projected
  arc A10 (537.35, 134) -> (531, 134) centre (534.175, 134) ccw projected
  line L20 (537.35, 134) -> (572, 134) projected
  line L21 (572, 134) -> (572, 168.65) projected
  arc A11 (572, 175) -> (572, 168.65) centre (572, 171.825) ccw projected
  line L22 (572, 175) -> (590, 175) projected
  line L23 (590, 175) -> (590, 208.3333) projected
  line L24 (590, 208.3333) -> (572, 208.3333) projected
  line L25 (572, 208.3333) -> (572, 291.6667) projected
  line L26 (572, 291.6667) -> (590, 291.6667) projected
  line L27 (590, 291.6667) -> (590, 375) projected
  line L28 (590, 375) -> (246.6667, 375) projected
  line L29 (246.6667, 375) -> (246.6667, 357) projected
  arc A12 (240.3167, 357) -> (246.6667, 357) centre (243.4917, 357) ccw projected
  line L30 (240.3167, 357) -> (205.6667, 357) projected
  line L31 (205.6667, 357) -> (205.6667, 322.35) projected
  arc A13 (205.6667, 316) -> (205.6667, 322.35) centre (205.6667, 319.175) ccw projected
  line L32 (205.6667, 316) -> (187.6667, 316) projected
  arc A14 (187.6667, 322.35) -> (187.6667, 316) centre (187.6667, 319.175) ccw projected
  line L33 (187.6667, 322.35) -> (187.6667, 357) projected
  line L34 (187.6667, 357) -> (153.0167, 357) projected
  arc A15 (146.6667, 357) -> (153.0167, 357) centre (149.8417, 357) ccw projected
  line L35 (146.6667, 357) -> (146.6667, 375) projected
  line L36 (146.6667, 375) -> (-146.6667, 375) projected
  line L37 (-146.6667, 375) -> (-146.6667, 357) projected
  arc A16 (-153.0167, 357) -> (-146.6667, 357) centre (-149.8417, 357) ccw projected
  line L38 (-153.0167, 357) -> (-187.6667, 357) projected
  line L39 (-187.6667, 357) -> (-187.6667, 322.35) projected
  arc A17 (-187.6667, 316) -> (-187.6667, 322.35) centre (-187.6667, 319.175) ccw projected
  line L40 (-187.6667, 316) -> (-205.6667, 316) projected
  arc A18 (-205.6667, 322.35) -> (-205.6667, 316) centre (-205.6667, 319.175) ccw projected
  line L41 (-205.6667, 322.35) -> (-205.6667, 357) projected
  line L42 (-205.6667, 357) -> (-240.3167, 357) projected
  arc A19 (-246.6667, 357) -> (-240.3167, 357) centre (-243.4917, 357) ccw projected
  line L43 (-246.6667, 357) -> (-246.6667, 375) projected
  line L44 (-246.6667, 375) -> (-590, 375) projected
  line L45 (-590, 375) -> (-590, 291.6667) projected
  line L46 (-590, 291.6667) -> (-572, 291.6667) projected
  line L47 (-572, 291.6667) -> (-572, 208.3333) projected
  line L48 (-572, 208.3333) -> (-590, 208.3333) projected
  line L49 (-590, 208.3333) -> (-590, 175) projected
  line L50 (-590, 175) -> (-572, 175) projected
  arc A20 (-572, 168.65) -> (-572, 175) centre (-572, 171.825) ccw projected
  line L51 (-572, 168.65) -> (-572, 134) projected
  line L52 (-572, 134) -> (-537.35, 134) projected
  arc A21 (-531, 134) -> (-537.35, 134) centre (-534.175, 134) ccw projected
  line L53 (-531, 134) -> (-531, 116) projected
  arc A22 (-537.35, 116) -> (-531, 116) centre (-534.175, 116) ccw projected
  line L54 (-537.35, 116) -> (-572, 116) projected
  line L55 (-572, 116) -> (-572, 81.35) projected
  arc A23 (-572, 75) -> (-572, 81.35) centre (-572, 78.175) ccw projected
  line L56 (-572, 75) -> (-590, 75) projected
  line L57 (-590, 75) -> (-590, -75) projected
  line L58 (-590, -75) -> (-572, -75) projected
  arc A24 (-572, -81.35) -> (-572, -75) centre (-572, -78.175) ccw projected
  line L59 (-572, -81.35) -> (-572, -116) projected
  line L60 (-572, -116) -> (-537.35, -116) projected
  arc A25 (-531, -116) -> (-537.35, -116) centre (-534.175, -116) ccw projected
  line L61 (-531, -116) -> (-531, -134) projected
  arc A26 (-537.35, -134) -> (-531, -134) centre (-534.175, -134) ccw projected
  line L62 (-537.35, -134) -> (-572, -134) projected
  line L63 (-572, -134) -> (-572, -168.65) projected
  arc A27 (-572, -175) -> (-572, -168.65) centre (-572, -171.825) ccw projected
  line L64 (-572, -175) -> (-590, -175) projected
  line L65 (-590, -175) -> (-590, -375) projected
  line L66 (-590, -375) -> (-246.6667, -375) projected
  line L67 (-246.6667, -375) -> (-246.6667, -357) projected
  arc A28 (-240.3167, -357) -> (-246.6667, -357) centre (-243.4917, -357) ccw projected
  line L68 (-240.3167, -357) -> (-205.6667, -357) projected
  line L69 (-205.6667, -357) -> (-205.6667, -322.35) projected
  arc A29 (-205.6667, -316) -> (-205.6667, -322.35) centre (-205.6667, -319.175) ccw projected
  line L70 (-205.6667, -316) -> (-187.6667, -316) projected
  arc A30 (-187.6667, -322.35) -> (-187.6667, -316) centre (-187.6667, -319.175) ccw projected
  line L71 (-187.6667, -322.35) -> (-187.6667, -357) projected
  line L72 (-187.6667, -357) -> (-153.0167, -357) projected
  arc A31 (-146.6667, -357) -> (-153.0167, -357) centre (-149.8417, -357) ccw projected
  line L73 (-146.6667, -357) -> (-146.6667, -375) projected
  line L74 (-146.6667, -375) -> (146.6667, -375) projected
  line L75 (146.6667, -375) -> (146.6667, -357) projected
  line L76 (246.6667, -116) -> (246.6667, -134) projected
  line L77 (246.6667, -134) -> (205.6667, -134) projected
  line L78 (205.6667, -134) -> (205.6667, -175) projected
  line L79 (205.6667, -175) -> (187.6667, -175) projected
  line L80 (187.6667, -175) -> (187.6667, -134) projected
  line L81 (187.6667, -134) -> (146.6667, -134) projected
  line L82 (146.6667, -134) -> (146.6667, -116) projected
  line L83 (146.6667, -116) -> (187.6667, -116) projected
  line L84 (187.6667, -116) -> (187.6667, -75) projected
  line L85 (187.6667, -75) -> (205.6667, -75) projected
  line L86 (205.6667, -75) -> (205.6667, -116) projected
  line L87 (205.6667, -116) -> (246.6667, -116) projected
  line L88 (-246.6667, -134) -> (-246.6667, -116) projected
  line L89 (-246.6667, -116) -> (-205.6667, -116) projected
  line L90 (-205.6667, -116) -> (-205.6667, -75) projected
  line L91 (-205.6667, -75) -> (-187.6667, -75) projected
  line L92 (-187.6667, -75) -> (-187.6667, -116) projected
  line L93 (-187.6667, -116) -> (-146.6667, -116) projected
  line L94 (-146.6667, -116) -> (-146.6667, -134) projected
  line L95 (-146.6667, -134) -> (-187.6667, -134) projected
  line L96 (-187.6667, -134) -> (-187.6667, -175) projected
  line L97 (-187.6667, -175) -> (-205.6667, -175) projected
  line L98 (-205.6667, -175) -> (-205.6667, -134) projected
  line L99 (-205.6667, -134) -> (-246.6667, -134) projected
  line L100 (246.6667, 134) -> (246.6667, 116) projected
  line L101 (246.6667, 116) -> (205.6667, 116) projected
  line L102 (205.6667, 116) -> (205.6667, 75) projected
  line L103 (205.6667, 75) -> (187.6667, 75) projected
  line L104 (187.6667, 75) -> (187.6667, 116) projected
  line L105 (187.6667, 116) -> (146.6667, 116) projected
  line L106 (146.6667, 116) -> (146.6667, 134) projected
  line L107 (146.6667, 134) -> (187.6667, 134) projected
  line L108 (187.6667, 134) -> (187.6667, 175) projected
  line L109 (187.6667, 175) -> (205.6667, 175) projected
  line L110 (205.6667, 175) -> (205.6667, 134) projected
  line L111 (205.6667, 134) -> (246.6667, 134) projected
  line L112 (-205.6667, 75) -> (-205.6667, 116) projected
  line L113 (-205.6667, 116) -> (-246.6667, 116) projected
  line L114 (-246.6667, 116) -> (-246.6667, 134) projected
  line L115 (-246.6667, 134) -> (-205.6667, 134) projected
  line L116 (-205.6667, 134) -> (-205.6667, 175) projected
  line L117 (-205.6667, 175) -> (-187.6667, 175) projected
  line L118 (-187.6667, 175) -> (-187.6667, 134) projected
  line L119 (-187.6667, 134) -> (-146.6667, 134) projected
  line L120 (-146.6667, 134) -> (-146.6667, 116) projected
  line L121 (-146.6667, 116) -> (-187.6667, 116) projected
  line L122 (-187.6667, 116) -> (-187.6667, 75) projected
  line L123 (-187.6667, 75) -> (-205.6667, 75) projected
  line L124 (-336.7778, 208.3333) -> (-336.7778, 291.6667) projected
  line L125 (-336.7778, 291.6667) -> (-318.7778, 291.6667) projected
  line L126 (-318.7778, 291.6667) -> (-318.7778, 208.3333) projected
  line L127 (-318.7778, 208.3333) -> (-336.7778, 208.3333) projected
  line L128 (336.7778, 291.6667) -> (336.7778, 208.3333) projected
  line L129 (336.7778, 208.3333) -> (318.7778, 208.3333) projected
  line L130 (318.7778, 208.3333) -> (318.7778, 291.6667) projected
  line L131 (318.7778, 291.6667) -> (336.7778, 291.6667) projected
  point P0 (0, 0)
  point P1 (-572, 288.4917)
  dimension "d62" = 3.175
  constraints: 1 vertical alignment
  measures "d62" distance from line of point (-572, 288.492) L46
hole "Hole3" at (-572, 18, -288.4917) direction (0, -1, 0) diameter 6.35 depth 9 tip angle 118
ref_plane "Work Plane6" through (-590, 9, -250) normal (0, 0, 1) x (1, 0, 0)
mirror "Mirror17" about plane through (-590, 9, -250) normal (0, 0, 1) of "Hole3"
mirror "Mirror18" about plane through (0, 0, 375) normal (-1, 0, 0) of "Hole3", "Mirror17"
sketch "Sketch14" plane through (0, 18, 0) normal (0, 1, 0) x (1, 0, 0)
  line L0 (336.7778, 291.6667) -> (336.7778, 208.3333) projected
  line L1 (336.7778, 208.3333) -> (318.7778, 208.3333) projected
  line L2 (318.7778, 208.3333) -> (318.7778, 291.6667) projected
  line L3 (318.7778, 291.6667) -> (336.7778, 291.6667) projected
  line L4 (-336.7778, 208.3333) -> (-336.7778, 291.6667) projected
  line L5 (-336.7778, 291.6667) -> (-318.7778, 291.6667) projected
  line L6 (-318.7778, 291.6667) -> (-318.7778, 208.3333) projected
  line L7 (-318.7778, 208.3333) -> (-336.7778, 208.3333) projected
  line L8 (-205.6667, 75) -> (-205.6667, 116) projected
  line L9 (-205.6667, 116) -> (-246.6667, 116) projected
  line L10 (-246.6667, 116) -> (-246.6667, 134) projected
  line L11 (-246.6667, 134) -> (-205.6667, 134) projected
  line L12 (-205.6667, 134) -> (-205.6667, 175) projected
  line L13 (-205.6667, 175) -> (-187.6667, 175) projected
  line L14 (-187.6667, 175) -> (-187.6667, 134) projected
  line L15 (-187.6667, 134) -> (-146.6667, 134) projected
  line L16 (-146.6667, 134) -> (-146.6667, 116) projected
  line L17 (-146.6667, 116) -> (-187.6667, 116) projected
  line L18 (-187.6667, 116) -> (-187.6667, 75) projected
  line L19 (-187.6667, 75) -> (-205.6667, 75) projected
  line L20 (246.6667, 134) -> (246.6667, 116) projected
  line L21 (246.6667, 116) -> (205.6667, 116) projected
  line L22 (205.6667, 116) -> (205.6667, 75) projected
  line L23 (205.6667, 75) -> (187.6667, 75) projected
  line L24 (187.6667, 75) -> (187.6667, 116) projected
  line L25 (187.6667, 116) -> (146.6667, 116) projected
  line L26 (146.6667, 116) -> (146.6667, 134) projected
  line L27 (146.6667, 134) -> (187.6667, 134) projected
  line L28 (187.6667, 134) -> (187.6667, 175) projected
  line L29 (187.6667, 175) -> (205.6667, 175) projected
  line L30 (205.6667, 175) -> (205.6667, 134) projected
  line L31 (205.6667, 134) -> (246.6667, 134) projected
  line L32 (-246.6667, -134) -> (-246.6667, -116) projected
  line L33 (-246.6667, -116) -> (-205.6667, -116) projected
  line L34 (-205.6667, -116) -> (-205.6667, -75) projected
  line L35 (-205.6667, -75) -> (-187.6667, -75) projected
  line L36 (-187.6667, -75) -> (-187.6667, -116) projected
  line L37 (-187.6667, -116) -> (-146.6667, -116) projected
  line L38 (-146.6667, -116) -> (-146.6667, -134) projected
  line L39 (-146.6667, -134) -> (-187.6667, -134) projected
  line L40 (-187.6667, -134) -> (-187.6667, -175) projected
  line L41 (-187.6667, -175) -> (-205.6667, -175) projected
  line L42 (-205.6667, -175) -> (-205.6667, -134) projected
  line L43 (-205.6667, -134) -> (-246.6667, -134) projected
  line L44 (246.6667, -116) -> (246.6667, -134) projected
  line L45 (246.6667, -134) -> (205.6667, -134) projected
  line L46 (205.6667, -134) -> (205.6667, -175) projected
  line L47 (205.6667, -175) -> (187.6667, -175) projected
  line L48 (187.6667, -175) -> (187.6667, -134) projected
  line L49 (187.6667, -134) -> (146.6667, -134) projected
  line L50 (146.6667, -134) -> (146.6667, -116) projected
  line L51 (146.6667, -116) -> (187.6667, -116) projected
  line L52 (187.6667, -116) -> (187.6667, -75) projected
  line L53 (187.6667, -75) -> (205.6667, -75) projected
  line L54 (205.6667, -75) -> (205.6667, -116) projected
  line L55 (205.6667, -116) -> (246.6667, -116) projected
  arc A0 (572, 214.6833) -> (572, 208.3333) centre (572, 211.5083) ccw projected
  line L56 (572, 214.6833) -> (572, 285.3167) projected
  arc A1 (572, 291.6667) -> (572, 285.3167) centre (572, 288.4917) ccw projected
  line L57 (572, 291.6667) -> (590, 291.6667) projected
  line L58 (590, 291.6667) -> (590, 375) projected
  line L59 (590, 375) -> (246.6667, 375) projected
  line L60 (246.6667, 375) -> (246.6667, 357) projected
  arc A2 (240.3167, 357) -> (246.6667, 357) centre (243.4917, 357) ccw projected
  line L61 (240.3167, 357) -> (205.6667, 357) projected
  line L62 (205.6667, 357) -> (205.6667, 322.35) projected
  arc A3 (205.6667, 316) -> (205.6667, 322.35) centre (205.6667, 319.175) ccw projected
  line L63 (205.6667, 316) -> (187.6667, 316) projected
  arc A4 (187.6667, 322.35) -> (187.6667, 316) centre (187.6667, 319.175) ccw projected
  line L64 (187.6667, 322.35) -> (187.6667, 357) projected
  line L65 (187.6667, 357) -> (153.0167, 357) projected
  arc A5 (146.6667, 357) -> (153.0167, 357) centre (149.8417, 357) ccw projected
  line L66 (146.6667, 357) -> (146.6667, 375) projected
  line L67 (146.6667, 375) -> (-146.6667, 375) projected
  line L68 (-146.6667, 375) -> (-146.6667, 357) projected
  arc A6 (-153.0167, 357) -> (-146.6667, 357) centre (-149.8417, 357) ccw projected
  line L69 (-153.0167, 357) -> (-187.6667, 357) projected
  line L70 (-187.6667, 357) -> (-187.6667, 322.35) projected
  arc A7 (-187.6667, 316) -> (-187.6667, 322.35) centre (-187.6667, 319.175) ccw projected
  line L71 (-187.6667, 316) -> (-205.6667, 316) projected
  arc A8 (-205.6667, 322.35) -> (-205.6667, 316) centre (-205.6667, 319.175) ccw projected
  line L72 (-205.6667, 322.35) -> (-205.6667, 357) projected
  line L73 (-205.6667, 357) -> (-240.3167, 357) projected
  arc A9 (-246.6667, 357) -> (-240.3167, 357) centre (-243.4917, 357) ccw projected
  line L74 (-246.6667, 357) -> (-246.6667, 375) projected
  line L75 (-246.6667, 375) -> (-590, 375) projected
  line L76 (-590, 375) -> (-590, 291.6667) projected
  line L77 (-590, 291.6667) -> (-572, 291.6667) projected
  arc A10 (-572, 285.3167) -> (-572, 291.6667) centre (-572, 288.4917) ccw projected
  line L78 (-572, 285.3167) -> (-572, 214.6833) projected
  arc A11 (-572, 208.3333) -> (-572, 214.6833) centre (-572, 211.5083) ccw projected
  line L79 (-572, 208.3333) -> (-590, 208.3333) projected
  line L80 (-590, 208.3333) -> (-590, 175) projected
  line L81 (-590, 175) -> (-572, 175) projected
  arc A12 (-572, 168.65) -> (-572, 175) centre (-572, 171.825) ccw projected
  line L82 (-572, 168.65) -> (-572, 134) projected
  line L83 (-572, 134) -> (-537.35, 134) projected
  arc A13 (-531, 134) -> (-537.35, 134) centre (-534.175, 134) ccw projected
  line L84 (-531, 134) -> (-531, 116) projected
  arc A14 (-537.35, 116) -> (-531, 116) centre (-534.175, 116) ccw projected
  line L85 (-537.35, 116) -> (-572, 116) projected
  line L86 (-572, 116) -> (-572, 81.35) projected
  arc A15 (-572, 75) -> (-572, 81.35) centre (-572, 78.175) ccw projected
  line L87 (-572, 75) -> (-590, 75) projected
  line L88 (-590, 75) -> (-590, -75) projected
  line L89 (-590, -75) -> (-572, -75) projected
  arc A16 (-572, -81.35) -> (-572, -75) centre (-572, -78.175) ccw projected
  line L90 (-572, -81.35) -> (-572, -116) projected
  line L91 (-572, -116) -> (-537.35, -116) projected
  arc A17 (-531, -116) -> (-537.35, -116) centre (-534.175, -116) ccw projected
  line L92 (-531, -116) -> (-531, -134) projected
  arc A18 (-537.35, -134) -> (-531, -134) centre (-534.175, -134) ccw projected
  line L93 (-537.35, -134) -> (-572, -134) projected
  line L94 (-572, -134) -> (-572, -168.65) projected
  arc A19 (-572, -175) -> (-572, -168.65) centre (-572, -171.825) ccw projected
  line L95 (-572, -175) -> (-590, -175) projected
  line L96 (-590, -175) -> (-590, -375) projected
  line L97 (-590, -375) -> (-246.6667, -375) projected
  line L98 (-246.6667, -375) -> (-246.6667, -357) projected
  arc A20 (-240.3167, -357) -> (-246.6667, -357) centre (-243.4917, -357) ccw projected
  line L99 (-240.3167, -357) -> (-205.6667, -357) projected
  line L100 (-205.6667, -357) -> (-205.6667, -322.35) projected
  arc A21 (-205.6667, -316) -> (-205.6667, -322.35) centre (-205.6667, -319.175) ccw projected
  line L101 (-205.6667, -316) -> (-187.6667, -316) projected
  arc A22 (-187.6667, -322.35) -> (-187.6667, -316) centre (-187.6667, -319.175) ccw projected
  line L102 (-187.6667, -322.35) -> (-187.6667, -357) projected
  line L103 (-187.6667, -357) -> (-153.0167, -357) projected
  arc A23 (-146.6667, -357) -> (-153.0167, -357) centre (-149.8417, -357) ccw projected
  line L104 (-146.6667, -357) -> (-146.6667, -375) projected
  line L105 (-146.6667, -375) -> (146.6667, -375) projected
  line L106 (146.6667, -375) -> (146.6667, -357) projected
  arc A24 (153.0167, -357) -> (146.6667, -357) centre (149.8417, -357) ccw projected
  line L107 (153.0167, -357) -> (187.6667, -357) projected
  line L108 (187.6667, -357) -> (187.6667, -322.35) projected
  arc A25 (187.6667, -316) -> (187.6667, -322.35) centre (187.6667, -319.175) ccw projected
  line L109 (187.6667, -316) -> (205.6667, -316) projected
  arc A26 (205.6667, -322.35) -> (205.6667, -316) centre (205.6667, -319.175) ccw projected
  line L110 (205.6667, -322.35) -> (205.6667, -357) projected
  line L111 (205.6667, -357) -> (240.3167, -357) projected
  arc A27 (246.6667, -357) -> (240.3167, -357) centre (243.4917, -357) ccw projected
  line L112 (246.6667, -357) -> (246.6667, -375) projected
  line L113 (246.6667, -375) -> (590, -375) projected
  line L114 (590, -375) -> (590, -175) projected
  line L115 (590, -175) -> (572, -175) projected
  arc A28 (572, -168.65) -> (572, -175) centre (572, -171.825) ccw projected
  line L116 (572, -168.65) -> (572, -134) projected
  line L117 (572, -134) -> (537.35, -134) projected
  arc A29 (531, -134) -> (537.35, -134) centre (534.175, -134) ccw projected
  line L118 (531, -134) -> (531, -116) projected
  arc A30 (537.35, -116) -> (531, -116) centre (534.175, -116) ccw projected
  line L119 (537.35, -116) -> (572, -116) projected
  line L120 (572, -116) -> (572, -81.35) projected
  arc A31 (572, -75) -> (572, -81.35) centre (572, -78.175) ccw projected
  line L121 (572, -75) -> (590, -75) projected
  line L122 (590, -75) -> (590, 75) projected
  line L123 (590, 75) -> (572, 75) projected
  arc A32 (572, 81.35) -> (572, 75) centre (572, 78.175) ccw projected
  line L124 (572, 81.35) -> (572, 116) projected
  line L125 (572, 116) -> (537.35, 116) projected
  arc A33 (531, 116) -> (537.35, 116) centre (534.175, 116) ccw projected
  line L126 (531, 116) -> (531, 134) projected
  arc A34 (537.35, 134) -> (531, 134) centre (534.175, 134) ccw projected
  line L127 (537.35, 134) -> (572, 134) projected
  line L128 (572, 134) -> (572, 168.65) projected
  arc A35 (572, 175) -> (572, 168.65) centre (572, 171.825) ccw projected
  line L129 (572, 175) -> (590, 175) projected
  line L130 (590, 175) -> (590, 208.3333) projected
  line L131 (590, 208.3333) -> (572, 208.3333) projected
  line L132 (-336.7778, 291.6667) -> (-318.7778, 291.6667) projected
  point P0 (0, 0)
  point P1 (-333.6028, 291.6667)
  point P2 (-327.7778, 291.6667)
  point P3 (-321.9528, 291.6667)
  point P4 (-327.7778, 291.6667)
  dimension "d70" = 3.175
  dimension "d71" = 3.175
  constraints: 2 horizontal alignment, 2 midpoint
  measures "d70" distance from line of L4 point (-333.603, 291.667)
  measures "d71" distance from line of L6 point (-321.953, 291.667)
hole "Hole4" at (-333.6028, 18, -291.6667) at (-321.9528, 18, -291.6667) direction (0, -1, 0) diameter 6.35 depth 9 tip angle 118
mirror "Mirror19" about plane through (-590, 9, -250) normal (0, 0, 1) of "Hole4"
mirror "Mirror20" about plane through (0, 0, 375) normal (-1, 0, 0) of "Hole4", "Mirror19"